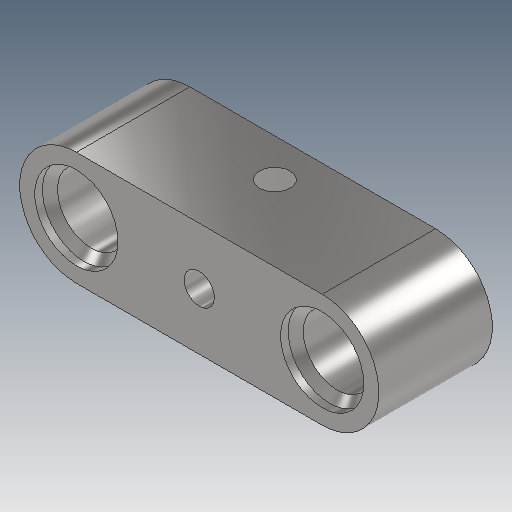
# Autodesk Inventor part: P2 lmao fila
Saved by Autodesk Inventor 2022 (Build 260153000, 153)
## iProperties
Created: 2021-11-07
Part Number: P2 lmao fila
Material: Ocel
Document SubType Name: Modeling
Designer: Jan Peřina
Density: 7.85 g/cm^3
Appearance: Pololeštěná
Stock Number: 3-G53-2/18
Mass: 483.118 g
Surface Area: 155.449 cm^2
Volume: 61.5437 cm^3
Author: Jan Peřina
Autodesk Inventor part; units mm, degrees
ref_plane "YZ Plane" through (0, 0, 0) normal (1, 0, 0) x (0, 1, 0)
ref_plane "XZ Plane" through (0, 0, 0) normal (0, 1, 0) x (-1, 0, 0)
ref_plane "XY Plane" through (0, 0, 0) normal (0, 0, 1) x (1, 0, 0)
sketch "Náčrt1" plane through (0, 0, 0) normal (0, 0, 1) x (1, 0, 0)
  line L0 (-32.5, -15) -> (32.5, -15)
  line L1 (47.5, 0) -> (47.5, 0)
  line L2 (32.5, 15) -> (-32.5, 15)
  line L3 (-47.5, 0) -> (-47.5, 0)
  line L4 (-47.5, -15) -> (47.5, 15) construction
  line L5 (47.5, -15) -> (-47.5, 15) construction
  arc A0 (-32.5, 15) -> (-47.5, 0) centre (-32.5, 0) ccw
  arc A1 (-47.5, 0) -> (-32.5, -15) centre (-32.5, 0) ccw
  arc A2 (32.5, -15) -> (47.5, 0) centre (32.5, 0) ccw
  arc A3 (47.5, 0) -> (32.5, 15) centre (32.5, 0) ccw
  point P0 (0, 0)
  point P1 (47.5, 0)
  point P2 (-47.5, 0)
  dimension "d0" = 95
  dimension "d1" = 30
  dimension "d2" = 15
  constraints: 12 end point, 8 point on circle, 8 point on line, 8 tangent, 4 centre point, 3 equal radius, 2 midpoint, 2 parallel, 1 horizontal, 1 perpendicular
  measures "d0" distance of L5.end L4.end
  measures "d1" distance of L4.end L5.start
  measures "d2" radius of A0
extrude "Vysunutí1" add sketch "Náčrt1" along normal blind 30
sketch "Náčrt2" plane through (0, 0, 30) normal (0, 0, 1) x (1, 0, 0)
  arc A0 (32.5, -15) -> (32.5, 15) centre (32.5, 0) ccw projected
  line L0 (32.5, 15) -> (-32.5, 15) projected
  arc A1 (-32.5, 15) -> (-32.5, -15) centre (-32.5, 0) ccw projected
  line L1 (-32.5, -15) -> (32.5, -15) projected
  point P0 (0, 0)
  constraints: 2 coincident, 2 horizontal alignment
hole "Díra1" at (-32.5, 0, 30) at (32.5, 0, 30) direction (0, 0, -1) diameter 15 end through all
sketch "Náčrt3" plane through (0, 0, 30) normal (0, 0, 1) x (1, 0, 0)
  circle A0 centre (-32.5, 0) radius 7.5 projected
  circle A1 centre (32.5, 0) radius 7.5 projected
  circle A2 centre (-32.5, 0) radius 11
  circle A3 centre (32.5, 0) radius 11
  point P0 (0, 0)
  dimension "d14" = 22
  dimension "d15" = 22
  constraints: 2 centre point, 2 coincident
  measures "d14" diameter of A2
  measures "d15" diameter of A3
extrude "Vysunutí2" cut sketch "Náčrt3" against normal blind 2 contours A1 | A2 | A3
sketch "Náčrt4" plane through (-32.5, 0, 28) normal (0, 0, 1) x (1, 0, 0)
  circle A0 centre (0, 0) radius 11 projected
  circle A1 centre (0, 0) radius 7.5 projected
  circle A2 centre (65, 0) radius 7.5 projected
  circle A3 centre (0, 0) radius 9
  circle A4 centre (65, 0) radius 9
  point P0 (32.5, 0)
  dimension "d18" = 18
  dimension "d19" = 18
  constraints: 2 centre point, 2 coincident
  measures "d18" diameter of A3
  measures "d19" diameter of A4
extrude "Vysunutí3" cut sketch "Náčrt4" against normal blind 17 contours A3 | A4
sketch "Náčrt5" plane through (0, 0, 0) normal (0, 0, -1) x (-1, 0, 0)
  circle A0 centre (32.5, 0) radius 7.5 projected
  circle A1 centre (-32.5, 0) radius 7.5 projected
  circle A2 centre (32.5, 0) radius 9
  circle A3 centre (-32.5, 0) radius 9
  point P0 (0, 0)
  dimension "d22" = 18
  dimension "d23" = 18
  constraints: 2 centre point, 2 coincident
  measures "d22" diameter of A2
  measures "d23" diameter of A3
extrude "Vysunutí4" cut sketch "Náčrt5" against normal blind 10
chamfer "Zkosení1" distance 2 angle 45 4 edges at (-23.5, 0, 0) (41.5, 0, 0) (-41.5, 0, 28) (23.5, 0, 28)
sketch "Náčrt6" plane through (0, 0, 30) normal (0, 0, 1) x (1, 0, 0)
  circle A0 centre (0, 0) radius 4
  dimension "d29" = 8
  constraints: 1 centre point, 1 coincident
  measures "d29" diameter of A0
extrude "Vysunutí5" cut sketch "Náčrt6" against normal blind 23
sketch "Náčrt7" plane through (-32.5, -15, 0) normal (0, -1, 0) x (1, 0, 0)
  circle A0 centre (32.5, 10) radius 4
  line L0 (0, 30) -> (65, 30) projected
  line L1 (0, 0) -> (65, 0) projected
  point P0 (32.5, 0)
  point P1 (32.5, 0)
  dimension "d32" = 8
  dimension "d33" = 20
  constraints: 1 centre point, 1 midpoint, 1 vertical alignment
  measures "d32" diameter of A0
  measures "d33" distance from line of L0 A0.centre
extrude "Vysunutí6" cut sketch "Náčrt7" against normal blind 9
mirror "Zrcadlit1" about plane through (0, 0, 0) normal (0, 1, 0) of "Vysunutí6"
